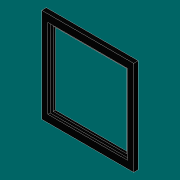
# Autodesk Inventor part: mirrorBackFrame
Saved by Autodesk Inventor 2016 (Build 200138000, 138)
## iProperties
Created: 2015-12-22
Part Number: mirrorBackFrame
Material: ABS Plastic
Document SubType Name: Modeling
Designer: sawai
Density: 1.06 g/cm^3
Appearance: Smooth - Black
Author: sawai
Autodesk Inventor part; units mm, degrees
ref_plane "YZ Plane" through (0, 0, 0) normal (1, 0, 0) x (0, 1, 0)
ref_plane "XZ Plane" through (0, 0, 0) normal (0, 1, 0) x (-1, 0, 0)
ref_plane "XY Plane" through (0, 0, 0) normal (0, 0, 1) x (1, 0, 0)
sketch "Sketch1" plane through (0, 0, 0) normal (0, 0, 1) x (1, 0, 0)
  line L0 (-57.15, 57.15) -> (57.15, 57.15) projected
  line L1 (57.15, 57.15) -> (57.15, -57.15) projected
  line L2 (57.15, -57.15) -> (-57.15, -57.15) projected
  line L3 (-57.15, -57.15) -> (-57.15, 57.15) projected
  line L4 (-63.3984, -63.5) -> (63.3984, -63.5) projected
  line L5 (63.3984, -63.5) -> (63.3984, 63.5) projected
  line L6 (63.3984, 63.5) -> (-63.3984, 63.5) projected
  line L7 (-63.3984, 63.5) -> (-63.3984, -63.5) projected
  point P0 (0, 0)
extrude "Extrusion1" add sketch "Sketch1" along normal blind 6.35 contours L0 L1 L2 L3 | L7 L6 L5 L4
sketch "Sketch2" plane through (0, 0, 6.35) normal (0, 0, 1) x (1, 0, 0)
  line L0 (50.9, 50.9) -> (-50.9, 50.9) projected
  line L1 (50.9, -50.9) -> (50.9, 50.9) projected
  line L2 (-50.9, -50.9) -> (50.9, -50.9) projected
  line L3 (-50.9, 50.9) -> (-50.9, -50.9) projected
  line L4 (-54.8688, 54.8688) -> (54.8688, 54.8688)
  line L5 (54.8688, 54.8688) -> (54.8688, -54.8688)
  line L6 (54.8688, -54.8688) -> (-54.8688, -54.8688)
  line L7 (-54.8688, -54.8688) -> (-54.8688, 54.8688)
  point P0 (0, 0)
  dimension "d2" = 3.9688
  constraints: 8 end point, 3 other
  measures "d2" distance between parallel lines of L0 L4
extrude "Extrusion2" cut sketch "Sketch2" against normal blind 3.175 contours L1 L2 L3 L0 | L4 L5 L6 L7
sketch "Sketch3" plane through (0, 0, 3.175) normal (0, 0, 1) x (1, 0, 0)
  line L0 (50.9, 50.9) -> (-50.9, 50.9) projected
  line L1 (-50.9, 50.9) -> (-50.9, -50.9) projected
  line L2 (50.9, -50.9) -> (50.9, 50.9) projected
  line L3 (-50.9, -50.9) -> (50.9, -50.9) projected
  point P0 (0, 0)
extrude "Extrusion3" cut sketch "Sketch3" against normal through all
sketch "Sketch4" plane through (0, 0, 6.35) normal (0, 0, 1) x (1, 0, 0)
  line L0 (-63.5, -65.0875) -> (63.5, -65.0875)
  line L1 (63.5, -65.0875) -> (63.5, 65.0875)
  line L2 (63.5, 65.0875) -> (-63.5, 65.0875)
  line L3 (-63.5, 65.0875) -> (-63.5, -65.0875)
  line L4 (-63.5, -65.0875) -> (63.5, 65.0875) construction
  line L5 (63.5, -65.0875) -> (-63.5, 65.0875) construction
  line L6 (-54.8688, -54.8688) -> (-54.8688, 54.8688) projected
  line L7 (-54.8688, 54.8688) -> (54.8688, 54.8688) projected
  line L8 (54.8688, 54.8688) -> (54.8688, -54.8688) projected
  line L9 (54.8688, -54.8688) -> (-54.8688, -54.8688) projected
  line L10 (-63.3984, -63.5) -> (63.3984, -63.5) projected
  line L11 (63.3984, -63.5) -> (63.3984, 63.5) projected
  line L12 (63.3984, 63.5) -> (-63.3984, 63.5) projected
  line L13 (-63.3984, 63.5) -> (-63.3984, -63.5) projected
  point P0 (0, 0)
  dimension "d7" = 130.175
  dimension "d8" = 127
  constraints: 12 end point, 2 midpoint, 2 parallel, 1 horizontal, 1 perpendicular
  measures "d7" distance of L0.end L1.end
  measures "d8" distance of L1.end L2.end
extrude "Extrusion4" add sketch "Sketch4" against normal up to surface (6.35 mm away) contours L3 L2 L1 L0
sketch "Sketch5" plane through (0, 0, 6.35) normal (0, 0, 1) x (1, 0, 0)
  line L0 (63.5, 65.0875) -> (-63.5, 65.0875) projected
  line L1 (-63.3984, -65.0875) -> (63.3984, -65.0875)
  line L2 (63.3984, -65.0875) -> (63.3984, 65.0875)
  line L3 (63.3984, 65.0875) -> (-63.3984, 65.0875)
  line L4 (-63.3984, 65.0875) -> (-63.3984, -65.0875)
  line L5 (-63.3984, -65.0875) -> (63.3984, 65.0875) construction
  line L6 (63.3984, -65.0875) -> (-63.3984, 65.0875) construction
  point P0 (0, 0)
  dimension "d11" = 126.7968
  constraints: 12 end point, 2 midpoint, 2 parallel, 1 horizontal, 1 perpendicular, 1 point on line
  measures "d11" distance between parallel lines of L4 L2
extrude "Extrusion5" cut sketch "Sketch5" against normal through all keep common part
equation "\"d0\" = plasticThickness"
equation "\"d2\" = 1.25 * mirrorThickness"
equation "\"d3\" = 0.5 * plasticThickness"
equation "\"d5\" = 0.5 * internalAcrylicThickness"
equation "\"d7\" = height + 2 * alignmentGrooveDepth"
equation "\"d8\" = width"
equation "\"d11\" = width - 2 * alignmentGrooveClearance"
equation "\"frameAcrylicThickness\" = 9.525"
equation "\"internalAcrylicThickness\" = 6.35"
equation "\"height\" = 127"
equation "\"width\" = 127"
equation "\"depth\" = 114.3"
equation "\"mirrorAngle\" = 5deg"
equation "\"detectorWidth\" = 52"
equation "\"detectorHeight\" = 52"
equation "\"mirrorThickness\" = 3.175"
equation "\"fresnelThickness\" = 0.254"
equation "\"focalLength\" = 76.2"
equation "\"ior\" = 1.49"
equation "\"centerThickness\" = 1.27"
equation "\"fresnelAngle\" = 90deg"
equation "\"fresnelEffectiveDiameter\" = 152.4"
equation "\"oRingWidth\" = 1.5875"
equation "\"sensorHolderDepth\" = 19.05"
equation "\"aerogelClearence\" = 3.175"
equation "\"backplanePCBWidth\" = 76.2"
equation "\"backplanePCBHeight\" = 76.2"
equation "\"backplaneHoleOffsett\" = 6.35"
equation "\"backplanePostionOffsett\" = 12.7"
equation "\"moduleSlotClearence\" = 0.79375"
equation "\"plasticThickness\" = 6.35"
equation "\"aerogelHolderDepth\" = 36.5125"
equation "\"caseThickness\" = 6.35"
equation "\"alignmentGrooveDepth\" = 1.5875"
equation "\"alignmentGrooveClearance\" = 0.1016"
equation "\"frontPanelThickness\" = 2.38125"
body "Solid1"
